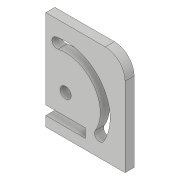
# Autodesk Inventor part: Angleframe
Saved by Autodesk Inventor 2017 (Build 210142000, 142)
## iProperties
Created: 2019-06-13
Part Number: Angleframe
Material: Generic
Document SubType Name: Modeling
Designer: markg
Density: 1 g/cm^3
Appearance: Default
Author: markg
Autodesk Inventor part; units mm, degrees
ref_plane "YZ Plane" through (0, 0, 0) normal (1, 0, 0) x (0, 1, 0)
ref_plane "XZ Plane" through (0, 0, 0) normal (0, 1, 0) x (-1, 0, 0)
ref_plane "XY Plane" through (0, 0, 0) normal (0, 0, 1) x (1, 0, 0)
sketch "Sketch1" plane through (0, 0, 0) normal (0, 0, 1) x (1, 0, 0)
  line L0 (0, 0) -> (25.4, 0)
  line L1 (25.4, 0) -> (25.4, 31.75)
  line L2 (25.4, 31.75) -> (0, 31.75)
  line L3 (0, 31.75) -> (0, 0)
  circle A0 centre (6.35, 12.7) radius 1.7882
  arc A1 (16.2884, 4.7932) -> (2.0063, 24.6341) centre (6.35, 12.7) ccw construction
  line L4 (2.5493, 23.1423) -> (1.4634, 26.1259)
  line L5 (6.35, 12.7) -> (20.6125, 12.7) construction
  arc A2 (15.0461, 5.7815) -> (2.5493, 23.1423) centre (6.35, 12.7) ccw
  arc A3 (17.5307, 3.8048) -> (1.4634, 26.1259) centre (6.35, 12.7) ccw
  line L6 (15.0461, 5.7815) -> (17.5307, 3.8048)
  dimension "d0" = 12.7
  dimension "d1" = 31.75
  dimension "d2" = 6.35
  dimension "d3" = 110
  dimension "d4" = 25.4
  dimension "d5" = 1.5875
  dimension "d6" = 1.5875
  dimension "d10" = 25.4
  constraints: 14 end point, 6 point on circle, 4 centre point, 2 coincident, 2 horizontal, 2 midpoint, 2 parallel, 1 perpendicular
  measures "d0" distance from line of L0 A0.centre
  measures "d1" distance of L2.end L0.start
  measures "d2" distance from line of A0.centre L3
  measures "d3" angle of L5 L4
  measures "d4" diameter of A1
  measures "d5" radial gap between concentric circles of A1 A2
  measures "d6" radial gap between concentric circles of A1 A3
  measures "d10" distance of L1.end L2.end
extrude "Extrusion1" add sketch "Sketch1" along normal blind 2.921
fillet "Fillet1" radius 1.5875 4 edges at (15.0461, 5.7815, 1.4605) (17.5307, 3.8048, 1.4605) (1.4634, 26.1259, 1.4605) (2.5493, 23.1423, 1.4605)
sketch "Sketch2" plane through (0, 0, 2.921) normal (0, 0, 1) x (1, 0, 0)
  line L0 (0, 3.175) -> (12.7, 3.175)
  line L1 (12.7, 3.175) -> (12.7, 6.096)
  line L2 (12.7, 6.096) -> (0, 6.096)
  line L3 (0, 6.096) -> (0, 3.175)
  line L4 (0, 0) -> (25.4, 0) projected
  line L5 (0, 31.75) -> (0, 0) projected
  dimension "d11" = 2.921
  dimension "d12" = 12.7
  dimension "d13" = 3.175
  dimension "d14" = 0
  constraints: 8 end point, 2 parallel, 1 horizontal, 1 perpendicular
  measures "d11" distance of L0.end L1.end
  measures "d12" distance of L1.end L2.end
  measures "d13" distance between parallel lines of L4 L0
  measures "d14" distance between parallel lines of L5 L3
extrude "Extrusion2" cut sketch "Sketch2" against normal blind 6.604
fillet "Fillet2" radius 6.35 1 edges at (25.4, 31.75, 1.4605)
body "Solid1"
